Autodesk Fusion 360 part; units mm, degrees
(part 6 of 6)
  spline S47 degree 5 poles (75.5315, 18.3528) (75.5386, 18.3616) (75.5527, 18.3792) (75.5738, 18.4056) (75.6017, 18.4408) (75.6365, 18.485) (75.671, 18.5292) (75.7053, 18.5736) (75.7393, 18.618) (75.7731, 18.6626) (75.8067, 18.7072) (75.84, 18.7519) (75.8731, 18.7967) (75.9059, 18.8417) (75.9385, 18.8867) (75.9708, 18.9318) (76.0029, 18.9769) (76.0347, 19.0222) (76.0663, 19.0676) (76.0976, 19.1131) (76.1287, 19.1586) (76.1595, 19.2043) (76.19, 19.25) (76.2203, 19.2958) (76.2503, 19.3417) (76.28, 19.3877) (76.3095, 19.4338) (76.3387, 19.48) (76.3676, 19.5263) (76.3962, 19.5726) (76.4246, 19.6191) (76.4527, 19.6656) (76.4804, 19.7122) (76.5079, 19.759) (76.5351, 19.8058) (76.562, 19.8526) (76.5886, 19.8996) (76.6149, 19.9467) (76.6409, 19.9938) (76.6666, 20.0411) (76.6919, 20.0884) (76.717, 20.1358) (76.7417, 20.1833) (76.766, 20.2309) (76.7901, 20.2786) (76.8138, 20.3264) (76.8371, 20.3742) (76.8602, 20.4221) (76.8828, 20.4702) (76.9051, 20.5183) (76.9271, 20.5665) (76.9486, 20.6148) (76.9697, 20.6632) (76.9904, 20.7116) (77.0107, 20.7602) (77.0306, 20.8089) (77.0501, 20.8576) (77.0693, 20.9064) (77.0881, 20.9553) (77.1064, 21.0043) (77.1241, 21.0534) (77.1413, 21.1027) (77.1577, 21.152) (77.1735, 21.2015) (77.1887, 21.2511) (77.2034, 21.3007) (77.2179, 21.3504) (77.232, 21.4002) (77.2456, 21.45) (77.2583, 21.5) (77.2696, 21.5501) (77.2771, 21.5905) (77.2817, 21.621) (77.2842, 21.6414) (77.2853, 21.6516) knots -1 -1 -1 -1 -1 -1 -0.98571429 -0.97142857 -0.95714286 -0.94285714 -0.92857143 -0.91428571 -0.9 -0.88571429 -0.87142857 -0.85714286 -0.84285714 -0.82857143 -0.81428571 -0.8 -0.78571429 -0.77142857 -0.75714286 -0.74285714 -0.72857143 -0.71428571 -0.7 -0.68571429 -0.67142857 -0.65714286 -0.64285714 -0.62857143 -0.61428571 -0.6 -0.58571429 -0.57142857 -0.55714286 -0.54285714 -0.52857143 -0.51428571 -0.5 -0.48571429 -0.47142857 -0.45714286 -0.44285714 -0.42857143 -0.41428571 -0.4 -0.38571429 -0.37142857 -0.35714286 -0.34285714 -0.32857143 -0.31428571 -0.3 -0.28571429 -0.27142857 -0.25714286 -0.24285714 -0.22857143 -0.21428571 -0.2 -0.18571429 -0.17142857 -0.15714286 -0.14285714 -0.12857143 -0.11428571 -0.1 -0.08571429 -0.07142857 -0.05714286 -0.04285714 -0.02857143 -0.01428571 0 0 0 0 0 0
  line L49 (77.2853, 21.6516) -> (77.3408, 22.1467)
  arc A101 (77.8821, 22.5891) -> (77.3408, 22.1467) centre (77.8377, 22.091) ccw
  circle A102 centre (79.882, 45) radius 22.5
  circle A103 centre (79.882, 45) radius 27
  line L50 (52.8825, 45.1611) -> (79.882, 45)
  circle A104 centre (79.882, 45) radius 20
  circle A105 centre (79.882, 45) radius 5
  circle A106 centre (79.882, 45) radius 7.5
  dimension "d9" = 40
  dimension "d10" = 15
  dimension "d11" = 10
  constraint concentric A0 A102
  constraint coincident A54.end A102
  constraint concentric A102 A103
  constraint coincident S20.end A103
  constraint coincident A103 L50.start
  constraint coincident A0.centre A2.centre
  constraint concentric A103 A104
  constraint concentric A104 A105
  constraint concentric A105 A106
  measures "d9" diameter of A104
  measures "d10" diameter of A106
  measures "d11" diameter of A105
extrude "Extruir6" cut sketch "Boceto6" against normal up to surface (3 mm away) contours S35 L37 A77 A78 A102 A103 L50 | A75 L36 S34 A76 S35 L37 A77 A102 A103 | S33 L35 A73 A74 A75 L36 S34 A102 A103 | A71 L34 S32 A72 S33 L35 A73 A102 A103 | S31 L33 A69 A70 A71 L34 S32 A102 A103 | A67 L32 S30 A68 S31 L33 A69 A102 A103 | S29 L31 A65 A66 A67 L32 S30 A102 A103 | A63 L30 S28 A64 S29 L31 A65 A102 A103 | S27 L29 A61 A62 A63 L30 S28 A102 A103 | L19 A42 A43 L20 S18 A102 A103 | A59 L28 S26 A60 S27 L29 A61 A102 A103 | A43 L20 S18 A44 S19 L21 A45 A102 A103 | S25 L27 A57 A58 A59 L28 S26 A102 A103 | S19 L21 A45 A46 A47 L22 S20 A102 A103 | A55 L26 S24 A56 S25 L27 A57 A102 A103 | A47 L22 S20 A48 S21 L23 A49 A102 A103 | S23 L25 A53 A54 A55 L26 S24 A102 A103 | S21 L23 A49 A50 A51 L24 S22 A102 A103 | A51 L24 S22 A52 S23 L25 A53 A102 A103
extrude "Extruir7" add sketch "Boceto6" along normal blind 1 contours A2 A6 A10 A14 A18 A22 A26 A30 A34 A38 A42 A46 A50 A54 A58 A62 A66 A70 A74 A78 A82 A86 A90 A94 A98 A102 | A106
move_body "Desplazar4" bodies 1 to x (1, 0, 0) y (0, 1, 0) z (0, 0, 1) at (-3, -79.882, -45)
move_body "Desplazar5" bodies 1 to x (1, 0, 0) y (0, -0.428935, 0.903335) z (0, -0.903335, -0.428935) at (0, 0, 0)
hole "Agujero1" at (0, 0, 0) direction (-1, 0, 0) diameter 3 depth 14 tip angle 180 counterbore diameter 5 counterbore depth 2
hole "Agujero2" at (0, -39.4047, 15.4425) direction (-1, 0, 0) diameter 3 depth 14 tip angle 180 counterbore diameter 5 counterbore depth 2
sketch "Boceto7" plane through (0, 0, 0) normal (1, 0, 0) x (0, 1, 0)
  circle A0 centre (0, 0) radius 20
  circle A1 centre (0, 0) radius 7.5
  circle A2 centre (0, 0) radius 10.7689
  dimension "d22" = 7
  text T0 "EPLA   ARI" font "Arial Black" height 7 bold align centre spacing 1 along the path A2 letters at x, y, angle (-17.3098, 13.2832, 43.1849) (-5.6194, 21.0831, 5.6111) (8.1277, 20.2035, -30.5273) (18.5703, 11.5458, -68.1772) (21.567, -1.0626, -97.1515) (20.2686, -7.4462, -114.503) (17.1256, -13.1521, -131.8545) (10.6744, -19.0845, -160.8287) (-4.3138, -21.4371, 158.5744) (-15.7563, -14.7974, 128.1521)
  constraint concentric A0 A2
extrude "Extruir8" add sketch "Boceto7" along normal blind 1 text T0
equation "d23 = 'EPLA   ARI'"
named bodies: "Engranaje tracción 2"
